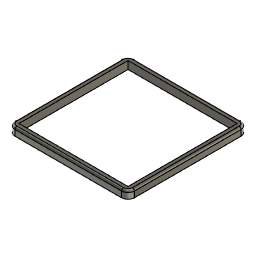
SolderingStation_TopBevel (Autodesk Fusion 360 design; units mm, degrees)
Autodesk Fusion 360 part; units mm, degrees
sketch "Sketch1" plane through (0, 0, 0) normal (0, 0, 1) x (1, 0, 0)
  line L0 (42.1, 42.1) -> (-42.1, 42.1)
  line L1 (-42.1, 42.1) -> (-42.1, -42.1)
  line L2 (-42.1, -42.1) -> (42.1, -42.1)
  line L3 (42.1, -42.1) -> (42.1, 42.1)
  line L4 (42.1, 42.1) -> (-42.1, -42.1) construction
  line L5 (-42.1, 42.1) -> (42.1, -42.1) construction
  line L6 (-46.1, -46.1) -> (46.1, -46.1)
  line L7 (46.1, -46.1) -> (46.1, 46.1)
  line L8 (46.1, 46.1) -> (-46.1, 46.1)
  line L9 (-46.1, 46.1) -> (-46.1, -46.1)
  dimension "d1" = 84.2
  dimension "d2" = 84.2
  dimension "d3" = 4
  constraint horizontal L0
  constraint perpendicular L0 L1
  constraint parallel L0 L2
  constraint parallel L1 L3
  constraint coincident L4 origin
  constraint coincident L5 origin
  measures "d1" distance of L1.end L2.end
  measures "d2" distance of L0.end L1.end
extrude "Extrude1" add sketch "Sketch1" along normal blind 6
fillet "Fillet1" radius 5 4 edges at (-46.1, -46.1, 3) (46.1, -46.1, 3) (46.1, 46.1, 3) (-46.1, 46.1, 3)
fillet "Fillet2" radius 1.5 8 edges at (-44.6355, 44.6355, 6) (-46.1, 0, 6) (-44.6355, -44.6355, 6) (0, -46.1, 6) (44.6355, -44.6355, 6) (46.1, 0, 6) (44.6355, 44.6355, 6) (0, 46.1, 6)
